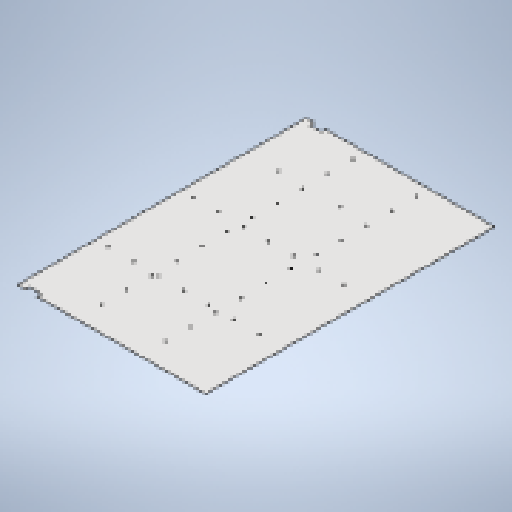
# Autodesk Inventor part: GnG frame 2 floor sheet 6
Saved by Autodesk Inventor 2025 (Build 290162010, 162A)
## iProperties
Created: 2025-10-28
Part Number: GnG frame 2 floor sheet 6
Material: Stainless Steel
Document SubType Name: Sheet Metal
Designer: admin
Mass: 280.619 g
Surface Area: 364.406 cm^2
Volume: 35.0774 cm^3
Density: 8 g/cm^3
Sheet Metal Rule: AISI304 3mm Die 32
Sheet Metal Width: 1500,000 mm
Sheet Metal Length: 2300,000 mm
Sheet Metal Area: 3450000,000 mm^2
Appearance: Default
Flat Pattern Width: 150 cm
Flat Pattern Length: 230 cm
Flat Pattern Area: 34500 cm^2
Author: admin
Autodesk Inventor part; units mm, degrees
ref_plane "YZ Plane" through (0, 0, 0) normal (1, 0, 0) x (0, 1, 0)
ref_plane "XZ Plane" through (0, 0, 0) normal (0, 1, 0) x (-1, 0, 0)
ref_plane "XY Plane" through (0, 0, 0) normal (0, 0, 1) x (1, 0, 0)
sketch "Sketch1" plane through (0, 0, 0) normal (0, 0, 1) x (1, 0, 0)
  line L0 (0, 0) -> (-1500, 0)
  line L1 (-1500, 0) -> (-1500, -2300)
  line L2 (-1500, -2300) -> (0, -2300)
  line L3 (0, -2300) -> (0, 0)
  line L4 (0, 0) -> (-30, 0)
  line L5 (-30, 0) -> (-30, -35)
  line L6 (-30, -35) -> (0, -35)
  line L7 (0, -35) -> (0, 0)
  line L8 (0, -2300) -> (-30, -2300)
  line L9 (-30, -2300) -> (-30, -2265)
  line L10 (-30, -2265) -> (0, -2265)
  line L11 (0, -2265) -> (0, -2300)
  line L12 (-1500, 0) -> (-1470, 0)
  line L13 (-1470, 0) -> (-1470, -35)
  line L14 (-1470, -35) -> (-1500, -35)
  line L15 (-1500, -35) -> (-1500, 0)
  line L16 (-1500, -2300) -> (-1470, -2300)
  line L17 (-1470, -2300) -> (-1470, -2265)
  line L18 (-1470, -2265) -> (-1500, -2265)
  line L19 (-1500, -2265) -> (-1500, -2300)
  line L20 (-1435, -2300) -> (-1345, -2300)
  line L21 (-1345, -2300) -> (-1345, -2265)
  line L22 (-1345, -2265) -> (-1435, -2265)
  line L23 (-1435, -2265) -> (-1435, -2300)
  line L24 (-1435, 0) -> (-1345, 0)
  line L25 (-1345, 0) -> (-1345, -35)
  line L26 (-1345, -35) -> (-1435, -35)
  line L27 (-1435, -35) -> (-1435, 0)
  point P0 (0, -35)
  point P1 (-30, 0)
  point P2 (0, -2265)
  point P3 (-1345, 0)
  point P4 (-1470, 0)
  point P5 (-1500, -35)
  point P6 (-1500, -2265)
  dimension "d22" = 1500
  dimension "d23" = 2300
  dimension "d24" = 30
  dimension "d25" = 35
  dimension "d28" = 90
  dimension "d41" = 65
  measures "d22" distance of L2.end L1.end
  measures "d23" distance of L1.end L0.end
  measures "d24" distance of L6.end L5.end
  measures "d25" distance of L5.end L4.end
  measures "d28" distance of L25.end L26.end
  measures "d41" distance between parallel lines of L27 L1
extrude "Plate1" add sketch "Sketch1" along normal blind 3 contours L3 L6 L5 L0 | L5 L6 L3 L10 L9 L2 L21 L22 L23 L17 L18 L1 L14 L13 L0 L27 L26 L25 | L3 L2 L9 L10 | L13 L14 L1 L0 | L18 L17 L2 L1
sketch "Sketch5" plane through (0, 0, 0) normal (0, 0, -1) x (-1, 0, 0)
  line L0 (1242.9543, 0) -> (1241.4294, -4.6556)
  arc A0 (1240.4791, -4.6556) -> (1241.4294, -4.6556) centre (1240.9543, -4.5) ccw
  line L1 (1240.4791, -4.6556) -> (1238.9543, 0)
  line L2 (1238.9543, 0) -> (1242.9543, 0)
  line L3 (1236.9543, 0) -> (1234.9543, 0)
  line L4 (1234.9543, 0) -> (1234.9543, -5)
  line L5 (1234.9543, -5) -> (1236.9543, -5)
  line L6 (1236.9543, -5) -> (1236.9543, 0)
  line L7 (1234.9543, 0) -> (1232.9543, 0) construction
  line L8 (1232.9543, 0) -> (1230.9543, 0)
  line L9 (1230.9543, 0) -> (1230.9543, -5)
  line L10 (1230.9543, -5) -> (1232.9543, -5)
  line L11 (1232.9543, -5) -> (1232.9543, 0)
  line L12 (1230.9543, 0) -> (1228.9543, 0) construction
  line L13 (1228.9543, 0) -> (1226.9543, 0)
  line L14 (1226.9543, 0) -> (1226.9543, -5)
  line L15 (1226.9543, -5) -> (1228.9543, -5)
  line L16 (1228.9543, -5) -> (1228.9543, 0)
  line L17 (1226.9543, 0) -> (1224.9543, 0) construction
  line L18 (1224.9543, 0) -> (1222.9543, 0)
  line L19 (1222.9543, 0) -> (1222.9543, -5)
  line L20 (1222.9543, -5) -> (1224.9543, -5)
  line L21 (1224.9543, -5) -> (1224.9543, 0)
  line L22 (1222.9543, 0) -> (1217.9543, 0) construction
  line L23 (1217.9543, 0) -> (1212.9543, 0) construction
  circle A1 centre (1217.9543, 0) radius 1
  circle A2 centre (1212.9543, 0) radius 1
  line L24 (0, 0) -> (1345, 0) projected
  point P0 (1240.9543, 0)
  dimension "d32" = 5
  dimension "d33" = 4
  dimension "d34" = 0.5
  dimension "d35" = 5
  dimension "d36" = 5
  dimension "d37" = 5
  dimension "d38" = 2
  constraints: 48 end point, 9 horizontal, 8 parallel, 5 equal length, 4 perpendicular, 3 centre point, 3 tangent, 2 coincident, 2 point on circle, 1 equal radius, 1 midpoint, 1 point on line, 1 vertical alignment
  measures "d32" distance of L4.end L4.start
  measures "d33" distance of L1.end L0.start
  measures "d34" radius of A0
  measures "d35" distance of L10.start L8.end
  measures "d36" distance of L14.end L14.start
  measures "d37" distance of L19.end L19.start
  measures "d38" diameter of A1
extrude "Cut1" cut sketch "Sketch5" against normal blind 3 contours L16 L15 L14 L13 | L21 L20 L19 L18 | L24 A1 | A1 L24 | L24 A2 | A2 L24
sketch "Sketch6" plane through (0, 0, 0) normal (0, 0, -1) x (-1, 0, 0)
  arc A0 (1211.9543, 0) -> (1213.9543, 0) centre (1212.9543, 0) ccw construction
  line L0 (0, 0) -> (1211.9543, 0) construction
  line L1 (0, -2300) -> (0, 0) construction
  line L2 (1345, -2300) -> (0, -2300) construction
  line L3 (1345, -2265) -> (1345, -2300) construction
  line L4 (1435, -2265) -> (1345, -2265) construction
  line L5 (1435, -2300) -> (1435, -2265) construction
  line L6 (1500, -2300) -> (1435, -2300) construction
  line L7 (1500, 0) -> (1500, -2300) construction
  line L8 (1435, 0) -> (1500, 0) construction
  line L9 (1435, -35) -> (1435, 0) construction
  line L10 (1345, -35) -> (1435, -35) construction
  line L11 (1345, 0) -> (1345, -35) construction
  line L12 (1228.9543, 0) -> (1345, 0) construction
  line L13 (1228.9543, 0) -> (1228.9543, -5) construction
  line L14 (1228.9543, -5) -> (1226.9543, -5) construction
  line L15 (1226.9543, -5) -> (1226.9543, 0) construction
  line L16 (1224.9543, 0) -> (1226.9543, 0) construction
  line L17 (1224.9543, 0) -> (1224.9543, -5) construction
  line L18 (1224.9543, -5) -> (1222.9543, -5) construction
  line L19 (1222.9543, -5) -> (1222.9543, 0) construction
  line L20 (1218.9543, 0) -> (1222.9543, 0) construction
  arc A1 (1216.9543, 0) -> (1218.9543, 0) centre (1217.9543, 0) ccw construction
  line L21 (1213.9543, 0) -> (1216.9543, 0) construction
  line L22 (1030, 0) -> (1030, -2300) construction
  line L23 (520, 0) -> (520, -2300) construction
  line L24 (0, -1675) -> (1500, -1675) construction
  line L25 (0, -1000) -> (1500, -1000) construction
  line L26 (1500, -475) -> (520, -475) construction
  circle A2 centre (1030, -2100) radius 7.5
  circle A3 centre (520, -2100) radius 7.5
  circle A4 centre (200, -1675) radius 7.5
  circle A5 centre (200, -1000) radius 7.5
  circle A6 centre (1030, -1900) radius 7.5
  circle A7 centre (520, -1900) radius 7.5
  circle A8 centre (1030, -1700) radius 7.5
  circle A9 centre (520, -1700) radius 7.5
  circle A10 centre (1030, -1500) radius 7.5
  circle A11 centre (520, -1500) radius 7.5
  circle A12 centre (1030, -1300) radius 7.5
  circle A13 centre (520, -1300) radius 7.5
  circle A14 centre (1030, -1100) radius 7.5
  circle A15 centre (520, -1100) radius 7.5
  circle A16 centre (1030, -900) radius 7.5
  circle A17 centre (520, -900) radius 7.5
  circle A18 centre (1030, -700) radius 7.5
  circle A19 centre (520, -700) radius 7.5
  circle A20 centre (1030, -500) radius 7.5
  circle A21 centre (520, -500) radius 7.5
  circle A22 centre (1030, -300) radius 7.5
  circle A23 centre (520, -300) radius 7.5
  circle A24 centre (1030, -100) radius 7.5
  circle A25 centre (520, -100) radius 7.5
  circle A26 centre (400, -1000) radius 7.5
  circle A27 centre (400, -1675) radius 7.5
  circle A28 centre (600, -1000) radius 7.5
  circle A29 centre (600, -1675) radius 7.5
  circle A30 centre (800, -1000) radius 7.5
  circle A31 centre (800, -1675) radius 7.5
  circle A32 centre (1000, -1000) radius 7.5
  circle A33 centre (1000, -1675) radius 7.5
  circle A34 centre (1200, -1000) radius 7.5
  circle A35 centre (1200, -1675) radius 7.5
  circle A36 centre (1400, -1000) radius 7.5
  circle A37 centre (1400, -1675) radius 7.5
  circle A38 centre (750, -475) radius 7.5
  circle A39 centre (1250, -475) radius 7.5
  dimension "d42" = 520
  dimension "d43" = 1030
  dimension "d44" = 625
  dimension "d45" = 1300
  dimension "d46" = 1825
  dimension "d47" = 15
  dimension "d48" = 200
  dimension "d49" = 200
  dimension "d52" = 200
  dimension "d59" = 200
  dimension "d66" = 250
  dimension "d67" = 750
  constraints: 38 centre point, 16 point on line, 10 end point, 5 equal radius, 5 perpendicular, 1 horizontal, 1 horizontal alignment, 1 vertical, 1 vertical alignment, 64 other
  measures "d42" distance between parallel lines of L23 L1
  measures "d43" distance between parallel lines of L22 L1
  measures "d44" distance between parallel lines of L2 L24
  measures "d45" distance between parallel lines of L25 L2
  measures "d46" distance between parallel lines of L26 L2
  measures "d47" diameter of A2
  measures "d48" distance from line of L2 A2.centre
  measures "d49" distance from line of A4.centre L1
  measures "d52" distance of A2.centre A6.centre
  measures "d59" distance of A5.centre A26.centre
  measures "d66" distance from line of L7 A39.centre
  measures "d67" distance from line of L7 A38.centre
extrude "Cut2" cut sketch "Sketch6" against normal blind 3
equation "\"d33\" = 2 * d31"
equation "\"d34\" = 0.25 * d31"
equation "\"d38\" = d31"
equation "\"d39\" = Thickness"
equation "\"d52\" = d48"
equation "\"d59\" = d49"
equation "\"d64\" = Thickness"
equation "\"d2\" = Thickness"
equation "\"BendReliefWidth\" = Thickness"
equation "\"BendReliefDepth\" = 0.5 * Thickness"
equation "\"CornerReliefSize\" = 4 * Thickness"
equation "\"MinimumRemnant\" = 2 * Thickness"
equation "\"TransitionRadius\" = BendRadius"
equation "\"JacobiRadiusSize\" = BendRadius"
equation "\"GapSize\" = Thickness"
equation "\"d31\" = 2"
equation "\"Thickness\" = 3"
equation "\"BendRadius\" = 5"
body "Solid1"
